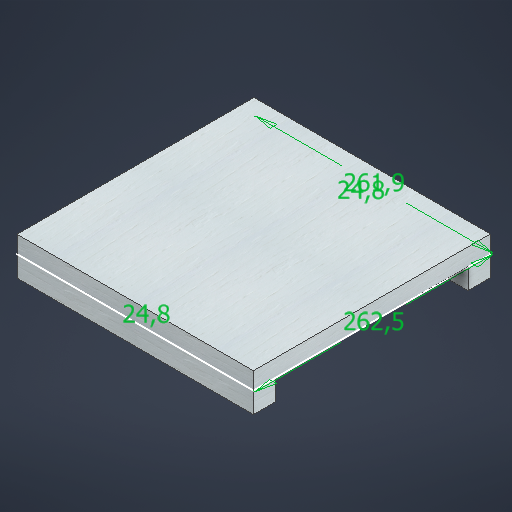
# Autodesk Inventor part: Tampa
Saved by Autodesk Inventor 2027 (Build 310192000, 192)
## iProperties
Created: 2026-10-01
Part Number: Tampa
Material: Genérico
Document SubType Name: Modeling
Designer: EspacoMaker
Density: 1 g/cm^3
Appearance: Padrão
Author: EspacoMaker
Autodesk Inventor part; units mm, degrees
ref_plane "YZ Plane" through (0, 0, 0) normal (1, 0, 0) x (0, 1, 0)
ref_plane "XZ Plane" through (0, 0, 0) normal (0, 1, 0) x (-1, 0, 0)
ref_plane "XY Plane" through (0, 0, 0) normal (0, 0, 1) x (1, 0, 0)
sketch "Esboço1" plane through (0, 0, 0) normal (0, 1, 0) x (-1, 0, 0)
  line L0 (130.95, 131.25) -> (-130.95, 131.25)
  line L1 (-130.95, 131.25) -> (-130.95, -131.25)
  line L2 (-130.95, -131.25) -> (130.95, -131.25)
  line L3 (130.95, -131.25) -> (130.95, 131.25)
  line L4 (130.95, 131.25) -> (-130.95, -131.25) construction
  line L5 (-130.95, 131.25) -> (130.95, -131.25) construction
  line L6 (130.95, 106.45) -> (-130.95, 106.45)
  line L7 (-130.95, -106.45) -> (130.95, -106.45)
  point P0 (0, 0)
  dimension "d0" = 261.9
  dimension "d1" = 262.5
  dimension "d2" = 24.8
  dimension "d3" = 24.8
  constraints: 16 end point, 4 parallel, 2 midpoint, 1 horizontal, 1 perpendicular
  measures "d0" distance of L2.end L1.end
  measures "d1" distance of L1.end L0.end
  measures "d2" distance between parallel lines of L0 L6
  measures "d3" distance between parallel lines of L2 L7
extrude "Extrusão1" add sketch "Esboço1" along normal blind 19
extrude "Extrusão2" add sketch "Esboço1" against normal blind 23 contours L3 L6 L1 L0 | L3 L2 L1 L7
